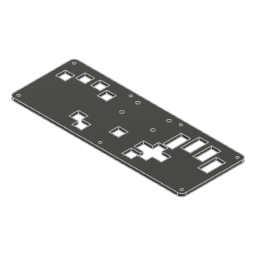
Top Panel Full (Autodesk Fusion 360 design; units mm, degrees)
Autodesk Fusion 360 part; units mm, degrees
sketch "Sketch1" plane through (0, 0, 0) normal (0, 0, 1) x (1, 0, 0)
  line L0 (89, 44) -> (69, 44)
  line L1 (43, -56) -> (63, -56)
  line L2 (-89, 24) -> (-69, 24)
  line L3 (-124, 33) -> (-124, 53)
  line L4 (-95, 36) -> (-95, 56)
  line L5 (174, 69) -> (-174, 69)
  line L6 (-174, -69) -> (174, -69)
  line L7 (170, 37) -> (150, 37)
  line L8 (150, 37) -> (150, -2)
  line L9 (-183, 60) -> (-183, -60)
  line L10 (-124, 53) -> (-144, 53)
  line L11 (115, 56) -> (95, 56)
  line L12 (-150, 37) -> (-170, 37)
  line L13 (-170, 37) -> (-170, 17)
  line L14 (-89, 44) -> (-89, 24)
  line L15 (-62, -36) -> (-62, -23)
  line L16 (-115, 36) -> (-95, 36)
  line L17 (-69, 24) -> (-69, 44)
  line L18 (-69, 44) -> (-89, 44)
  line L19 (-62, -23) -> (-82, -23)
  line L20 (124, 14) -> (144, 14)
  line L21 (-144, 33) -> (-124, 33)
  circle A0 centre (173, -59) radius 2.6
  line L22 (-10, -30) -> (10, -30)
  line L23 (82, -30) -> (101, -30)
  line L24 (-43, -56) -> (-43, -36)
  line L25 (-63, -43) -> (-63, -56)
  line L26 (-82, -43) -> (-63, -43)
  circle A1 centre (-173, -59) radius 2.6
  line L27 (-144, 53) -> (-144, 33)
  line L28 (-10, -10) -> (-10, -30)
  line L29 (-150, 17) -> (-150, 37)
  line L30 (-115, 56) -> (-115, 36)
  line L31 (-63, -56) -> (-43, -56)
  line L32 (-170, 17) -> (-150, 17)
  line L33 (82, 3) -> (62, 3)
  line L34 (115, 17) -> (115, 56)
  line L35 (43, -30) -> (62, -30)
  line L36 (170, -2) -> (170, 37)
  line L37 (95, 56) -> (95, 17)
  line L38 (63, -43) -> (82, -43)
  line L39 (89, 5) -> (89, 44)
  circle A2 centre (0, -59) radius 2.6
  line L40 (183, -60) -> (183, 60)
  circle A3 centre (-173, 59) radius 2.6
  line L41 (43, -36) -> (43, -56)
  line L42 (62, 3) -> (62, -10)
  line L43 (69, 44) -> (69, 5)
  line L44 (10, -10) -> (-10, -10)
  line L45 (43, -10) -> (43, -30)
  line L46 (101, -30) -> (101, -10)
  line L47 (144, 53) -> (124, 53)
  line L48 (62, -10) -> (43, -10)
  line L49 (82, -43) -> (82, -30)
  line L50 (-95, 56) -> (-115, 56)
  line L51 (-82, -23) -> (-82, -43)
  line L52 (124, 53) -> (124, 14)
  line L53 (150, -2) -> (170, -2)
  circle A4 centre (173, 59) radius 2.6
  line L54 (62, -30) -> (62, -36)
  line L55 (10, -30) -> (10, -10)
  line L56 (95, 17) -> (115, 17)
  line L57 (101, -10) -> (82, -10)
  line L58 (62, -36) -> (43, -36)
  line L59 (82, -10) -> (82, 3)
  line L60 (63, -56) -> (63, -43)
  line L61 (69, 5) -> (89, 5)
  line L62 (144, 14) -> (144, 53)
  line L63 (-43, -36) -> (-62, -36)
  arc A5 (-174, 69) -> (-183, 60) centre (-174, 60) ccw
  arc A6 (183, 60) -> (174, 69) centre (174, 60) ccw
  arc A7 (174, -69) -> (183, -60) centre (174, -60) ccw
  arc A8 (-183, -60) -> (-174, -69) centre (-174, -60) ccw
  circle A9 centre (33, 54) radius 3.5
  circle A10 centre (-33, 54) radius 3.5
  circle A11 centre (33, 20) radius 3.5
  circle A12 centre (-33, 20) radius 3.5
  circle A13 centre (53, 59) radius 2.6
  circle A14 centre (-53, 59) radius 2.6
  dimension "d1" = 9
  dimension "d2" = 7
  dimension "d3" = 7
  dimension "d4" = 7
  dimension "d5" = 7
  dimension "d8" = 5.2
  dimension "d9" = 5.2
  constraint vertical L9
  constraint vertical L40
  constraint horizontal L6
  constraint tangent L9 A5
  constraint tangent L5 A5
  constraint tangent L40 A6
  constraint tangent L5 A6
  constraint equal A5 A6
  constraint tangent L40 A7
  constraint tangent L6 A7
  constraint equal A5 A7
  constraint tangent L6 A8
  constraint tangent L9 A8
  constraint equal A5 A8
  measures "d1" radius of A5
  measures "d2" diameter of A9
  measures "d3" diameter of A10
  measures "d4" diameter of A11
  measures "d5" diameter of A12
  measures "d8" diameter of A13
  measures "d9" diameter of A14
extrude "Extrude1" add sketch "Sketch1" along normal blind 6
